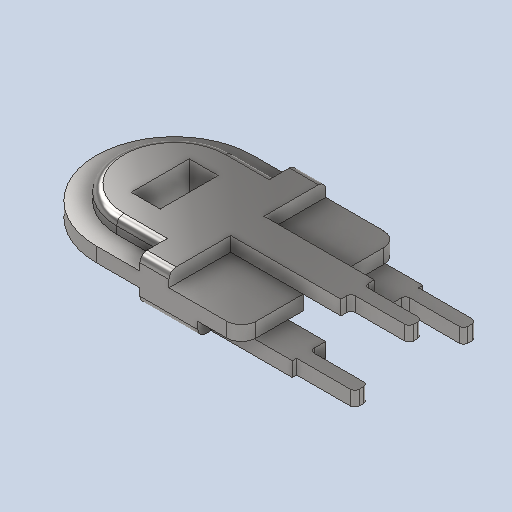
# Autodesk Inventor part: potencjometr
Saved by Autodesk Inventor 2024.2 (Build 282272000, 272)
## iProperties
Created: 2024-01-20
Part Number: potencjometr
Material: Stal nierdzewna
Document SubType Name: Modeling
Designer: Konrad
Density: 8 g/cm^3
Appearance: Częściowo polerowany
Author: Konrad
Autodesk Inventor part; units mm, degrees
ref_plane "YZ Plane" through (0, 0, 0) normal (1, 0, 0) x (0, 1, 0)
ref_plane "XZ Plane" through (0, 0, 0) normal (0, 1, 0) x (-1, 0, 0)
ref_plane "XY Plane" through (0, 0, 0) normal (0, 0, 1) x (1, 0, 0)
sketch "Szkic1" plane through (0, 0, 0) normal (0, 1, 0) x (-1, 0, 0)
  circle A0 centre (0, 0) radius 5.4 construction
  line L0 (-1, 2) -> (1, 2)
  line L1 (1, 2) -> (1, -2)
  line L2 (1, -2) -> (-1, -2)
  line L3 (-1, -2) -> (-1, 2)
  line L4 (-1, 2) -> (1, -2) construction
  line L5 (1, 2) -> (-1, -2) construction
  line L6 (0, -5.4) -> (0, 5.4)
  line L7 (0, 5.4) -> (-7, 5.4)
  line L8 (-7, 5.4) -> (-7, -5.4)
  line L9 (-7, -5.4) -> (0, -5.4)
  circle A1 centre (0, 0) radius 4 construction
  line L10 (-12.6, 4.5) -> (-12.6, 2.2)
  line L11 (-12.6, 2.2) -> (-7, 2.2)
  line L12 (-7, 2.2) -> (-7, 5.4)
  line L13 (-12.6, -4.5) -> (-12.6, -2.2)
  line L14 (-12.6, -2.2) -> (-7, -2.2)
  line L15 (-7, -2.2) -> (-7, -5.4)
  line L16 (-12.6, 4.2) -> (-16.6, 4.2)
  line L17 (-16.6, 4.2) -> (-16.6, 3.3)
  line L18 (-16.6, 3.3) -> (-12.6, 3.3)
  line L19 (-12.6, 3.3) -> (-12.6, 4.2)
  line L20 (-12.6, -4.2) -> (-16.6, -4.2)
  line L21 (-16.6, -4.2) -> (-16.6, -3.3)
  line L22 (-16.6, -3.3) -> (-12.6, -3.3)
  line L23 (-12.6, -3.3) -> (-12.6, -4.2)
  line L24 (-12.6, 1.15) -> (-7, 1.15)
  line L25 (-7, 1.15) -> (-7, -1.15)
  line L26 (-7, -1.15) -> (-12.6, -1.15)
  line L27 (-12.6, -1.15) -> (-12.6, 1.15)
  line L28 (-16.6, 0.45) -> (-12.6, 0.45)
  line L29 (-12.6, 0.45) -> (-12.6, -0.45)
  line L30 (-12.6, -0.45) -> (-16.6, -0.45)
  line L31 (-16.6, -0.45) -> (-16.6, 0.45)
  line L32 (-12.6, 2.2) -> (-12.6, 1.15) construction
  line L33 (-12.6, -1.15) -> (-12.6, -2.2) construction
  line L34 (9.8, 0) -> (-21, 0) construction
  line L35 (-12.6, 4.5) -> (-7, 4.5)
  line L36 (-12.6, -4.5) -> (-7, -4.5)
  line L37 (-7, 5.4) -> (-10, 5.4)
  line L38 (-10, 5.4) -> (-10, -5.4)
  line L39 (-10, -5.4) -> (-7, -5.4)
  line L40 (-3, 5.4) -> (-3, -5.4)
  line L41 (-7, 1.15) -> (-3, 1.15)
  line L42 (-7, -1.15) -> (-3, -1.15)
  line L43 (-5, 5.4) -> (-5, -5.4)
  arc A2 (0, -5.4) -> (0, 5.4) centre (0, 0) ccw
  arc A3 (0, -4) -> (0, 4) centre (0, 0) ccw
  line L44 (0, -4) -> (-3, -4)
  line L45 (0, 4) -> (-3, 4)
  point P0 (-10, 4.5)
  point P1 (-10, -4.5)
  point P2 (-5, 1.15)
  point P3 (0, 4)
  point P4 (-5, -1.15)
  point P5 (-10, -1.15)
  point P6 (-10, 1.15)
  dimension "d0" = 10.8
  dimension "d1" = 18
  dimension "d2" = 4
  dimension "d3" = 0.9
  dimension "d4" = 7.5
  dimension "d5" = 2.3
  dimension "d6" = 0.3
  dimension "d7" = 3
  dimension "d8" = 2
  dimension "d9" = 8
  dimension "d10" = 3
  dimension "d11" = 2
  dimension "d12" = 4
  dimension "d13" = 2
  constraints: 91 end point, 20 point on line, 17 perpendicular, 15 parallel, 8 point on circle, 6 horizontal, 4 centre point, 4 coincident, 4 collinear, 3 midpoint, 2 vertical, 1 tangent, 5 other
  measures "d0" diameter of A0
  measures "d2" distance of L20.start L20.end
  measures "d3" distance of L20.end L21.end
  measures "d4" distance of L17.end L20.end
  measures "d5" distance between parallel lines of L26 L24
  measures "d6" distance between parallel lines of L16 L35
  measures "d7" distance of L38.end L8.end
  measures "d8" distance between parallel lines of L8 L43
  measures "d9" diameter of A1
  measures "d10" distance from line of point (0, 0) L40
  measures "d11" distance between parallel lines of L40 L43
  measures "d12" distance of L0.end L1.end
  measures "d13" distance of L0.start L0.end
extrude "Wyciągnięcie proste1" add sketch "Szkic1" along normal blind 1 contours L45 L40 L7 L6 | L6 A2 A3 | L6 L9 L40 L44 | L43 L41 L8 L7 | L9 L8 L42 L43 | L8 L35 L38 L37 | L24 L38 L11 L8 | L39 L38 L36 L8 | L8 L14 L38 L26 | L8 L11 L38 L35 | L36 L38 L14 L8
extrude "Wyciągnięcie proste2" add sketch "Szkic1" along normal blind 2 contours L3 L2 L6 L44 L40 L45 L0 | L6 A3 L2 L1 L0 | L40 L41 L43 L7 | L40 L9 L43 L42 | L40 L42 L43 L41 | L43 L42 L8 L41 | L8 L26 L38 L24 | L38 L26 L27 L24 | L27 L30 L31 L28
extrude "Wyciągnięcie proste3" cut sketch "Szkic1" along normal blind 1 contours L8 L26 L38 L24 | L38 L26 L27 L24 | L27 L30 L31 L28
extrude "Wyciągnięcie proste4" add sketch "Szkic1" against normal blind 1 contours L3 L2 L6 L44 L40 L45 L0 | L6 A3 L2 L1 L0 | L40 L41 L43 L7 | L40 L9 L43 L42 | L40 L42 L43 L41 | L43 L41 L8 L7 | L9 L8 L42 L43 | L8 L11 L38 L35 | L36 L38 L14 L8 | L38 L11 L10 L35 | L36 L13 L14 L38 | L10 L18 L17 L16 | L20 L21 L22 L13
fillet "Zaokrąglenie1" radius 0.3 10 edges at (16.6, 1.5, -0.45) (16.6, 1.5, 0.45) (16.6, -0.5, 3.3) (16.6, -0.5, 4.2) (16.6, -0.5, -3.3) (16.6, -0.5, -4.2) (12.6, -0.5, -3.3) (12.6, -0.5, 3.3) (12.6, 1.5, -0.45) (12.6, 1.5, 0.45)
fillet "Zaokrąglenie2" radius 1 2 edges at (10, 0.5, 5.4) (10, 0.5, -5.4)
fillet "Zaokrąglenie3" radius 0.5 10 edges at (4, 2, 5.4) (4, 2, -5.4) (-4, 2, 0) (1.5, 2, 4) (1.5, 2, -4) (5, -1, 5.4) (-4, -1, 0) (1.5, -1, -4) (1.5, -1, 4) (5, -1, -5.4)
